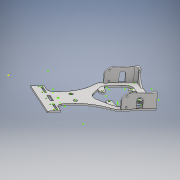
# Autodesk Inventor part: Khung_xe_ver2
Saved by Autodesk Inventor 2018.3 (Build 223284000, 284)
## iProperties
Created: 2018-09-22
Part Number: Khung_xe_ver2
Material: Generic
Document SubType Name: Modeling
Designer: lehoang
Density: 1 g/cm^3
Appearance: Default
Author: lehoang
## iProperties of the stored document Khung_xe_ver2_3DPrint.ipt
Created: 2018-09-22
Part Number: Khung_xe_ver2_3DPrint
Material: Generic
Document SubType Name: Modeling
Designer: lehoang
Density: 1 g/cm^3
Appearance: Default
Author: lehoang
Autodesk Inventor part; units mm, degrees
ref_plane "YZ Plane" through (0, 0, 0) normal (1, 0, 0) x (0, 1, 0)
ref_plane "XZ Plane" through (0, 0, 0) normal (0, 1, 0) x (-1, 0, 0)
ref_plane "XY Plane" through (0, 0, 0) normal (0, 0, 1) x (1, 0, 0)
sketch "Sketch1" plane through (0, 0, 0) normal (0, 0, 1) x (1, 0, 0)
  circle A0 centre (112.978, 33.5391) radius 1
  circle A1 centre (134.278, 33.5391) radius 1
  line L0 (38.778, 165.0391) -> (41.778, 165.0391)
  circle A2 centre (102.578, 73.9391) radius 3.2
  circle A3 centre (70.278, 123.0391) radius 1.6
  line L1 (80.278, 41.884) -> (80.278, 37.0391)
  line L2 (100.278, 41.884) -> (80.278, 41.884)
  line L3 (100.278, 37.0391) -> (100.278, 41.884)
  circle A4 centre (90.278, 33.5391) radius 1
  circle A5 centre (67.578, 33.5391) radius 1
  circle A6 centre (46.278, 33.5391) radius 1
  line L4 (138.778, 140.0391) -> (138.778, 132.0391)
  line L5 (41.778, 140.0391) -> (41.778, 132.5391)
  line L6 (138.778, 140.0391) -> (138.778, 155.0391)
  line L7 (132.078, 182.5391) -> (132.078, 185.5391)
  line L8 (133.778, 182.5391) -> (132.078, 182.5391)
  arc A7 (138.778, 177.5391) -> (133.778, 182.5391) centre (133.778, 177.5391) ccw
  line L9 (138.778, 177.5391) -> (138.778, 165.0391)
  line L10 (138.778, 155.0391) -> (141.778, 155.0391)
  line L11 (138.778, 165.0391) -> (138.778, 155.0391)
  line L12 (141.778, 165.0391) -> (138.778, 165.0391)
  line L13 (141.778, 160.0391) -> (138.778, 160.0391)
  line L14 (41.778, 140.0391) -> (41.778, 155.0391)
  line L15 (48.478, 182.5391) -> (48.478, 185.5391)
  line L16 (46.778, 182.5391) -> (48.478, 182.5391)
  arc A8 (46.778, 182.5391) -> (41.778, 177.5391) centre (46.778, 177.5391) ccw
  line L17 (41.778, 177.5391) -> (41.778, 165.0391)
  line L18 (41.778, 155.0391) -> (38.778, 155.0391)
  line L19 (41.778, 165.0391) -> (41.778, 155.0391)
  line L20 (38.778, 160.0391) -> (41.778, 160.0391)
  line L21 (138.778, 140.0391) -> (141.778, 140.0391)
  line L22 (38.778, 140.0391) -> (41.778, 140.0391)
  arc A9 (105.278, 167.0391) -> (103.8125, 172.5391) centre (94.1966, 167.0318) ccw
  arc A10 (116.7067, 172.4709) -> (115.278, 167.0391) centre (126.3343, 167.0349) ccw
  arc A11 (76.7434, 172.5391) -> (75.278, 167.0391) centre (86.3593, 167.0318) ccw
  arc A12 (65.278, 167.0391) -> (63.9569, 172.2715) centre (54.2558, 167.0391) ccw
  arc A13 (105.278, 167.0391) -> (115.278, 167.0391) centre (110.278, 167.0391) ccw
  arc A14 (65.278, 167.0391) -> (75.278, 167.0391) centre (70.278, 167.0391) ccw
  line L23 (100.278, 37.0391) -> (80.278, 37.0391)
  arc A15 (52.2389, 130.436) -> (70.278, 128.0391) centre (70.278, 197.1187) ccw
  arc A16 (70.278, 118.0391) -> (70.278, 128.0391) centre (70.278, 123.0391) ccw
  arc A17 (70.278, 118.0391) -> (63.8674, 117.741) centre (70.278, 48.9595) ccw
  arc A18 (117.5879, 117.6513) -> (110.278, 118.0391) centre (110.278, 48.9595) ccw
  arc A19 (110.278, 128.0391) -> (110.278, 118.0391) centre (110.278, 123.0391) ccw
  arc A20 (110.278, 128.0391) -> (129.8835, 130.8796) centre (110.278, 197.1187) ccw
  arc A21 (67.0393, 51.0617) -> (44.6359, 118.397) centre (-10.5277, 62.6486) ccw
  arc A22 (38.778, 132.5391) -> (44.6359, 118.397) centre (58.778, 132.5391) ccw
  line L24 (38.778, 132.5391) -> (38.778, 185.5391)
  line L25 (38.778, 185.5391) -> (141.778, 185.5391)
  line L26 (141.778, 185.5391) -> (141.778, 132.5391)
  arc A23 (135.9201, 118.397) -> (141.778, 132.5391) centre (121.778, 132.5391) ccw
  arc A24 (135.9201, 118.397) -> (113.5167, 51.0617) centre (191.0837, 62.6486) ccw
  arc A25 (113.5167, 51.0617) -> (123.4069, 42.5391) centre (123.4069, 52.5391) ccw
  line L27 (123.4069, 42.5391) -> (138.278, 42.5391)
  line L28 (138.278, 42.5391) -> (138.278, 22.5391)
  line L29 (138.278, 22.5391) -> (42.278, 22.5391)
  line L30 (42.278, 22.5391) -> (42.278, 42.5391)
  line L31 (42.278, 42.5391) -> (57.149, 42.5391)
  arc A26 (57.149, 42.5391) -> (67.0393, 51.0617) centre (57.149, 52.5391) ccw
  line L32 (47.278, 39.6391) -> (67.278, 39.6391)
  arc A27 (67.278, 36.4391) -> (67.278, 39.6391) centre (67.278, 38.0391) ccw
  line L33 (67.278, 36.4391) -> (47.278, 36.4391)
  arc A28 (47.278, 39.6391) -> (47.278, 36.4391) centre (47.278, 38.0391) ccw
  line L34 (133.278, 39.6391) -> (113.278, 39.6391)
  arc A29 (113.278, 39.6391) -> (113.278, 36.4391) centre (113.278, 38.0391) ccw
  line L35 (113.278, 36.4391) -> (133.278, 36.4391)
  arc A30 (133.278, 36.4391) -> (133.278, 39.6391) centre (133.278, 38.0391) ccw
  circle A31 centre (77.978, 73.9391) radius 3.2
  line L36 (78.8179, 106.9845) -> (58.0176, 121.9499)
  arc A32 (51.778, 134.1259) -> (58.0176, 121.9499) centre (66.778, 134.1259) ccw
  line L37 (51.778, 134.1259) -> (51.778, 157.5391)
  arc A33 (66.778, 172.5391) -> (51.778, 157.5391) centre (66.778, 157.5391) ccw
  line L38 (66.778, 172.5391) -> (115.278, 172.5391)
  arc A34 (130.278, 157.5391) -> (115.278, 172.5391) centre (115.278, 157.5391) ccw
  line L39 (130.278, 157.5391) -> (130.278, 134.2972)
  arc A35 (123.8177, 121.9654) -> (130.278, 134.2972) centre (115.278, 134.2972) ccw
  line L40 (123.8177, 121.9654) -> (101.8847, 106.7768)
  arc A36 (78.8179, 106.9845) -> (101.8847, 106.7768) centre (90.4984, 123.2192) ccw
  circle A37 centre (110.278, 123.0391) radius 1.6
  circle A38 centre (110.278, 167.0391) radius 1.6
  circle A39 centre (70.278, 167.0391) radius 1.6
  line L41 (38.778, 132.5391) -> (41.778, 132.5391)
  line L42 (138.778, 132.0391) -> (141.7717, 132.0391)
  circle A40 centre (90.278, 51.0617) radius 1.6
  point P0 (0, 0)
  constraints: 86 end point, 63 point on circle, 41 centre point, 14 point on line, 2 midpoint, 1 horizontal, 1 perpendicular
extrude "Đế" add sketch "Sketch1" against normal blind 3 contours L24 L25 L15 L16 A8 L17 L0 | L0 L19 L20 L24 | L17 A8 L16 L15 L25 L7 L8 A7 L9 L11 L6 L4 L42 A23 A24 A25 L27 L28 L29 L30 L31 A26 A21 A22 L41 L5 L14 L19 | L20 L19 L18 L24 | L18 L14 L22 L24 | L22 L5 L41 L24 | L25 L26 L12 L9 A7 L8 L7 | L26 L13 L11 L12 | L26 L10 L11 L13 | L26 L21 L6 L10 | L26 A23 L42 L4 L21 | A9 L38 A34 A10 A13 | A11 A14 A12 A33 L38 | A35 L40 A18 A19 A20 | A15 A16 A17 L36 A32
extrude "Giá ĐC" add sketch "Sketch1" along normal blind 24 contours L24 L25 L15 L16 A8 L17 L0 | L0 L19 L20 L24 | L20 L19 L18 L24 | L18 L14 L22 L24 | L22 L5 L41 L24 | L25 L26 L12 L9 A7 L8 L7 | L26 L13 L11 L12 | L26 L10 L11 L13 | L26 L21 L6 L10 | L26 A23 L42 L4 L21
fillet "Fillet1" radius 18.35 2 edges at (48.478, 184.0391, 0) (132.078, 184.0391, 0)
fillet "Fillet2" radius 12 2 edges at (40.278, 132.5391, 24) (140.2749, 132.0391, 24)
sketch "Sketch3" plane through (0, 0, -3) normal (0, 0, -1) x (-1, 0, 0)
  line L0 (-69.9726, 86.9521) -> (-111.3035, 86.9521) construction
  line L1 (-111.3035, 86.9521) -> (-111.3035, 94.8074) construction
  line L2 (-111.3035, 94.8074) -> (-69.9726, 94.8074) construction
  line L3 (-69.9726, 94.8074) -> (-69.9726, 86.9521) construction
  line L4 (-73.6405, 93.0521) -> (-70.3581, 93.0521)
  line L5 (-70.3581, 93.0521) -> (-70.3581, 91.9893)
  line L6 (-70.3581, 91.9893) -> (-71.2331, 91.9893)
  line L7 (-71.2331, 91.9893) -> (-71.2331, 88.0149)
  line L8 (-71.2331, 88.0149) -> (-70.3581, 88.0149)
  line L9 (-70.3581, 88.0149) -> (-70.3581, 86.9521)
  line L10 (-70.3581, 86.9521) -> (-73.6405, 86.9521)
  line L11 (-73.6405, 86.9521) -> (-73.6405, 88.0149)
  line L12 (-73.6405, 88.0149) -> (-72.7655, 88.0149)
  line L13 (-72.7655, 88.0149) -> (-72.7655, 91.9893)
  line L14 (-72.7655, 91.9893) -> (-73.6405, 91.9893)
  line L15 (-73.6405, 91.9893) -> (-73.6405, 93.0521)
  line L16 (-79.8838, 93.0521) -> (-78.4107, 93.0521)
  line L17 (-78.4107, 93.0521) -> (-76.0577, 88.8009)
  line L18 (-76.0577, 88.8009) -> (-76.0577, 93.0521)
  line L19 (-76.0577, 93.0521) -> (-74.6588, 93.0521)
  line L20 (-74.6588, 93.0521) -> (-74.6588, 86.9521)
  line L21 (-74.6588, 86.9521) -> (-76.5372, 86.9521)
  line L22 (-76.5372, 86.9521) -> (-78.4849, 90.447)
  line L23 (-78.4849, 90.447) -> (-78.4849, 86.9521)
  line L24 (-78.4849, 86.9521) -> (-79.8838, 86.9521)
  line L25 (-79.8838, 86.9521) -> (-79.8838, 93.0521)
  line L26 (-85.2077, 88.1138) -> (-82.6471, 88.1138)
  line L27 (-82.6471, 88.1138) -> (-82.6471, 89.2656)
  line L28 (-82.6471, 89.2656) -> (-85.0051, 89.2656)
  line L29 (-85.0051, 89.2656) -> (-85.0051, 90.4272)
  line L30 (-85.0051, 90.4272) -> (-82.6471, 90.4272)
  line L31 (-82.6471, 90.4272) -> (-82.6471, 93.0521)
  line L32 (-82.6471, 93.0521) -> (-81.1246, 93.0521)
  line L33 (-81.1246, 93.0521) -> (-81.1246, 86.9521)
  line L34 (-81.1246, 86.9521) -> (-85.2077, 86.9521)
  line L35 (-85.2077, 86.9521) -> (-85.2077, 88.1138)
  line L36 (-89.0338, 93.0521) -> (-85.7515, 93.0521)
  line L37 (-85.7515, 93.0521) -> (-85.7515, 91.9893)
  line L38 (-85.7515, 91.9893) -> (-86.6265, 91.9893)
  line L39 (-86.6265, 91.9893) -> (-86.6265, 88.0149)
  line L40 (-86.6265, 88.0149) -> (-85.7515, 88.0149)
  line L41 (-85.7515, 88.0149) -> (-85.7515, 86.9521)
  line L42 (-85.7515, 86.9521) -> (-89.0338, 86.9521)
  line L43 (-89.0338, 86.9521) -> (-89.0338, 88.0149)
  line L44 (-89.0338, 88.0149) -> (-88.1589, 88.0149)
  line L45 (-88.1589, 88.0149) -> (-88.1589, 91.9893)
  line L46 (-88.1589, 91.9893) -> (-89.0338, 91.9893)
  line L47 (-89.0338, 91.9893) -> (-89.0338, 93.0521)
  line L48 (-95.2772, 93.0521) -> (-93.8041, 93.0521)
  line L49 (-93.8041, 93.0521) -> (-91.4511, 88.8009)
  line L50 (-91.4511, 88.8009) -> (-91.4511, 93.0521)
  line L51 (-91.4511, 93.0521) -> (-90.0522, 93.0521)
  line L52 (-90.0522, 93.0521) -> (-90.0522, 86.9521)
  line L53 (-90.0522, 86.9521) -> (-91.9306, 86.9521)
  line L54 (-91.9306, 86.9521) -> (-93.8782, 90.447)
  line L55 (-93.8782, 90.447) -> (-93.8782, 86.9521)
  line L56 (-93.8782, 86.9521) -> (-95.2772, 86.9521)
  line L57 (-95.2772, 86.9521) -> (-95.2772, 93.0521)
  line L58 (-99.5531, 93.0521) -> (-96.2708, 93.0521)
  line L59 (-96.2708, 93.0521) -> (-96.2708, 91.9893)
  line L60 (-96.2708, 91.9893) -> (-97.1458, 91.9893)
  line L61 (-97.1458, 91.9893) -> (-97.1458, 88.0149)
  line L62 (-97.1458, 88.0149) -> (-96.2708, 88.0149)
  line L63 (-96.2708, 88.0149) -> (-96.2708, 86.9521)
  line L64 (-96.2708, 86.9521) -> (-99.5531, 86.9521)
  line L65 (-99.5531, 86.9521) -> (-99.5531, 88.0149)
  line L66 (-99.5531, 88.0149) -> (-98.6782, 88.0149)
  line L67 (-98.6782, 88.0149) -> (-98.6782, 91.9893)
  line L68 (-98.6782, 91.9893) -> (-99.5531, 91.9893)
  line L69 (-99.5531, 91.9893) -> (-99.5531, 93.0521)
  line L70 (-101.743, 93.0521) -> (-101.743, 88.1138)
  line L71 (-101.743, 88.1138) -> (-99.9387, 88.1138)
  line L72 (-99.9387, 88.1138) -> (-99.9387, 86.9521)
  line L73 (-99.9387, 86.9521) -> (-105.0797, 86.9521)
  line L74 (-105.0797, 86.9521) -> (-105.0797, 88.1138)
  line L75 (-105.0797, 88.1138) -> (-103.2754, 88.1138)
  line L76 (-103.2754, 88.1138) -> (-103.2754, 93.0521)
  line L77 (-103.2754, 93.0521) -> (-101.743, 93.0521)
  line L78 (-110.7793, 86.9521) -> (-108.6735, 90.5063)
  line L79 (-108.6735, 90.5063) -> (-108.6735, 93.0521)
  line L80 (-108.6735, 93.0521) -> (-107.1411, 93.0521)
  line L81 (-107.1411, 93.0521) -> (-107.1411, 90.5805)
  line L82 (-107.1411, 90.5805) -> (-105.0006, 86.9521)
  line L83 (-105.0006, 86.9521) -> (-106.7456, 86.9521)
  line L84 (-106.7456, 86.9521) -> (-107.9369, 89.1271)
  line L85 (-107.9369, 89.1271) -> (-109.0887, 86.9521)
  line L86 (-109.0887, 86.9521) -> (-110.7793, 86.9521)
  point P0 (0, 0)
  constraints: 2 other
extrude "Copyright" cut sketch "Sketch3" against normal blind 1
sketch "Sketch4" plane through (41.778, 132.5391, 0) normal (1, 0, 0) x (0, 0, -1)
  line L0 (0, 22.5002) -> (-13, 22.5002)
  line L1 (0, 32.5002) -> (-13, 32.5002)
  line L2 (0, 22.5002) -> (0, 32.5002)
  line L3 (-18, 27.5002) -> (-18, 27.5002)
  arc A0 (-18, 27.5002) -> (-13, 22.5002) centre (-13, 27.5002) ccw
  arc A1 (-13, 32.5002) -> (-18, 27.5002) centre (-13, 27.5002) ccw
  circle A2 centre (-3, 7.5) radius 1.6
  circle A3 centre (-20.2, 7.5) radius 1.6
  point P0 (0, -132.5391)
  constraints: 8 end point, 4 centre point, 4 point on circle, 4 tangent, 2 parallel, 1 concentric, 1 horizontal, 1 vertical
extrude "Extrusion5" cut sketch "Sketch4" along normal mid plane 230.6
fillet "Fillet3" radius 2.475 2 edges at (48.478, 184.0391, 24) (132.078, 184.0391, 24)
body "Solid1"
